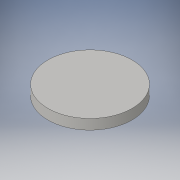
# Autodesk Inventor part: LED housing 2
Saved by Autodesk Inventor 2016 (Build 200138000, 138)
## iProperties
Created: 2017-09-27
Part Number: LED housing 2
Material: Generic
Document SubType Name: Modeling
Designer: Student
Density: 1 g/cm^3
Appearance: Default
Author: Student
Autodesk Inventor part; units mm, degrees
ref_plane "YZ Plane" through (0, 0, 0) normal (1, 0, 0) x (0, 1, 0)
ref_plane "XZ Plane" through (0, 0, 0) normal (0, 1, 0) x (-1, 0, 0)
ref_plane "XY Plane" through (0, 0, 0) normal (0, 0, 1) x (1, 0, 0)
sketch "Sketch1" plane through (0, 0, 0) normal (0, 1, 0) x (-1, 0, 0)
  circle A0 centre (0, 0) radius 31.75
  dimension "d0" = 63.5
  constraints: 1 centre point, 1 coincident
  measures "d0" diameter of A0
extrude "Extrusion1" add sketch "Sketch1" along normal blind 2.54
sketch "Sketch2" plane through (0, 0, 0) normal (0, -1, 0) x (1, 0, 0)
  circle A0 centre (0, 0) radius 31.75 projected
  circle A1 centre (0, 0) radius 17.018
  circle A2 centre (0, 0) radius 31.75
  dimension "d4" = 34.036
  constraints: 2 centre point, 2 coincident, 1 concentric
  measures "d4" diameter of A1
extrude "Extrusion2" add sketch "Sketch2" along normal blind 5.08
sketch "Sketch3" plane through (0, -5.08, 0) normal (0, -1, 0) x (1, 0, 0)
  circle A0 centre (0, 0) radius 23.495
  circle A1 centre (0, 0) radius 17.018 projected
  circle A2 centre (0, 0) radius 26.162
  dimension "d7" = 46.99
  dimension "d8" = 52.324
  constraints: 2 centre point, 2 coincident
  measures "d7" diameter of A0
  measures "d8" diameter of A2
extrude "Extrusion3" cut sketch "Sketch3" against normal blind 2.667 contours A2
sketch "Sketch5" plane through (0, -5.08, 0) normal (0, -1, 0) x (1, 0, 0)
  point P0 (0, 0)
  point P1 (-28.575, 0)
  point P2 (0, -28.575)
  point P3 (28.575, 0)
  point P4 (0, 28.575)
  dimension "d18" = 28.575
  dimension "d32" = 360
  constraints: 5 other
  measures "d18" distance of point (0, 0) point (-28.575, 0)
hole "Hole1" at (-28.575, -5.08, 0) at (0, -5.08, 28.575) at (28.575, -5.08, 0) at (0, -5.08, -28.575) direction (0, 1, 0) diameter 3 depth 1.27 tip angle 118
body "Solid1"
